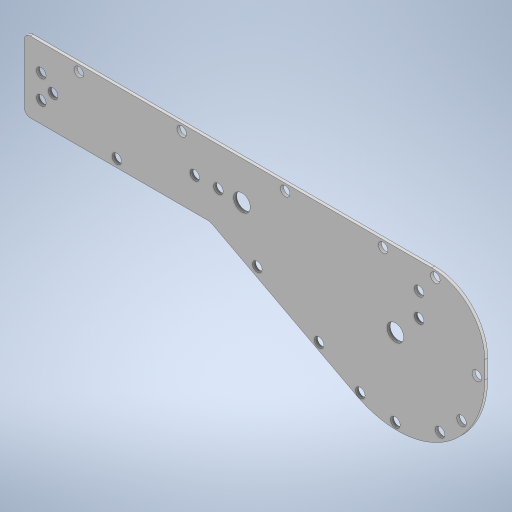
# Autodesk Inventor part: intake sled v5
Saved by Autodesk Inventor 2023.4 (Build 274418000, 418)
## iProperties
Created: 2023-12-16
Part Number: intake sled v5
Material: Generic
Document SubType Name: Modeling
Designer: Meer
Density: 1 g/cm^3
Appearance: Default
Author: Meer
Autodesk Inventor part; units mm, degrees
ref_plane "YZ Plane" through (0, 0, 0) normal (1, 0, 0) x (0, 1, 0)
ref_plane "XZ Plane" through (0, 0, 0) normal (0, 1, 0) x (-1, 0, 0)
ref_plane "XY Plane" through (0, 0, 0) normal (0, 0, 1) x (1, 0, 0)
sketch "Sketch1" plane through (0, 0, 0) normal (0, 0, 1) x (1, 0, 0)
  line L0 (0, 0) -> (247.65, 0)
  line L1 (247.65, 0) -> (247.65, 38.1)
  line L2 (247.65, 38.1) -> (0, 38.1)
  line L3 (0, 38.1) -> (0, 0)
  line L4 (286.1616, 0) -> (255.1962, 0)
  line L5 (255.1962, 0) -> (255.1962, 12.7)
  line L6 (255.1962, 12.7) -> (286.1616, 12.7)
  line L7 (286.1616, 12.7) -> (286.1616, 0)
  line L8 (247.65, 12.7) -> (200.66, 12.7)
  circle A0 centre (200.6294, 0) radius 47.0206
  line L9 (16.2468, 38.1) -> (16.2468, 12.7)
  line L10 (16.2468, 12.7) -> (155.3565, 12.7)
  line L11 (0, 12.7) -> (17.7951, 12.7)
  line L12 (179.5891, -42.0504) -> (75.8552, 12.7)
  point P0 (99.9175, 0)
  dimension "d0" = 247.65
  dimension "d1" = 38.1
  dimension "d2" = 12.7
  dimension "d3" = 30.9654
  dimension "d4" = 46.99
  dimension "d10" = 25.4
  constraints: 26 end point, 7 point on line, 5 perpendicular, 4 parallel, 3 point on circle, 2 horizontal, 1 centre point
  measures "d0" distance of L1.end L2.end
  measures "d1" distance of L0.end L1.end
  measures "d2" distance of L6.end L4.start
  measures "d3" distance of L5.end L6.end
  measures "d4" distance of L8.start L8.end
  measures "d10" distance of L9.start L9.end
extrude "Extrusion1" add sketch "Sketch1" along normal blind 1.5875 contours L3 L11 L10 L12 L0 | L12 L10 A0 L0 | L0 A0 L12 | L3 L2 L9 L11 | A0 L2 L0 | L0 A0 L12 | L10 L9 L2 A0 | A0 L8 L1 | L8 A0 L2 L1
fillet "Fillet1" radius 28.575 1 edges at (247.65, 38.1, 0.7937)
fillet "Fillet2" radius 3.175 1 edges at (0, 38.1, 0.7937)
fillet "Fillet4" radius 3.175 1 edges at (0, 0, 0.7937)
fillet "Fillet5" radius 5.08 1 edges at (99.9175, 0, 0.7937)
sketch "Sketch3" plane through (0, 0, 1.5875) normal (0, 0, 1) x (1, 0, 0)
  line L0 (9.1438, 0) -> (9.1438, 11.176)
  line L1 (9.1438, 11.176) -> (-0.0002, 11.176)
  circle A0 centre (9.1438, 11.176) radius 2.54
  line L2 (9.1438, 11.176) -> (9.1438, 23.876)
  circle A1 centre (9.1438, 23.876) radius 2.54
  line L3 (9.1438, 17.526) -> (15.4938, 17.526)
  circle A2 centre (15.4938, 17.526) radius 2.54
  line L4 (15.4938, 17.526) -> (91.6938, 17.526)
  circle A3 centre (91.6938, 17.526) radius 2.54
  line L5 (91.6938, 17.526) -> (104.3938, 17.526)
  circle A4 centre (104.3938, 17.526) radius 2.54
  line L6 (104.3938, 17.526) -> (117.0938, 17.526)
  circle A5 centre (117.0938, 17.526) radius 4.445
  line L7 (9.1438, 11.176) -> (212.3438, 11.176)
  line L8 (9.1438, 23.876) -> (212.3438, 23.876)
  circle A6 centre (212.3438, 23.876) radius 2.54
  circle A7 centre (212.3438, 11.176) radius 2.54
  circle A8 centre (125.3488, -8.3154) radius 2.54
  line L9 (125.3488, -8.3154) -> (158.5861, -26.9405)
  circle A9 centre (158.5861, -26.9405) radius 2.54
  line L10 (158.5861, -26.9405) -> (180.7442, -39.3573)
  circle A10 centre (180.7442, -39.3573) radius 2.54
  circle A11 centre (199.6056, -43.6188) radius 2.54
  circle A12 centre (223.6318, -36.189) radius 2.54
  circle A13 centre (235.2038, -25.0926) radius 2.54
  circle A14 centre (243.4585, 0) radius 2.54
  circle A15 centre (29.3464, 34.4582) radius 2.54
  circle A16 centre (84.6567, 34.4582) radius 2.54
  circle A17 centre (140.3584, 34.4582) radius 2.54
  circle A18 centre (192.9921, 34.4582) radius 2.54
  circle A19 centre (221.0918, 34.4582) radius 2.54
  circle A20 centre (49.7674, 4.225) radius 2.54
  arc A21 (101.0303, -0.5874) -> (98.6591, 0) centre (98.6591, -5.08) ccw projected
  line L11 (98.6591, 0) -> (199.6241, 0)
  line L12 (199.6241, 0) -> (199.6241, -1.778)
  circle A22 centre (199.6241, -1.778) radius 4.445
  point P0 (0, 0)
  point P1 (160.8019, -28.1822)
  point P2 (156.3703, -25.6989)
  point P3 (94.2338, 17.526)
  point P4 (89.1538, 17.526)
  point P5 (6.6038, 11.176)
  point P6 (9.1438, 8.636)
  point P7 (18.0338, 17.526)
  point P8 (12.9538, 17.526)
  point P9 (11.6838, 23.876)
  point P10 (9.1438, 21.336)
  dimension "d14" = 11.176
  dimension "d15" = 9.144
  dimension "d16" = 5.08
  dimension "d17" = 12.7
  dimension "d18" = 5.08
  dimension "d19" = 6.35
  dimension "d20" = 5.08
  dimension "d21" = 76.2
  dimension "d22" = 5.08
  dimension "d23" = 12.7
  dimension "d24" = 5.08
  dimension "d25" = 12.7
  dimension "d26" = 8.89
  dimension "d27" = 203.2
  dimension "d28" = 203.2
  dimension "d29" = 5.08
  dimension "d30" = 5.08
  dimension "d31" = 5.08
  dimension "d32" = 38.1
  dimension "d33" = 5.08
  dimension "d34" = 25.4
  dimension "d35" = 5.08
  dimension "d36" = 5.08
  dimension "d37" = 5.08
  dimension "d38" = 5.08
  dimension "d39" = 5.08
  dimension "d40" = 5.08
  dimension "d41" = 5.08
  dimension "d42" = 5.08
  dimension "d43" = 5.08
  dimension "d44" = 5.08
  dimension "d47" = 5.08
  dimension "d48" = 100.965
  dimension "d50" = 1.778
  dimension "d51" = 8.89
  constraints: 26 end point, 22 centre point, 12 coincident, 5 horizontal, 3 vertical, 2 point on line, 1 midpoint, 1 perpendicular
  measures "d14" distance of L0.start L0.end
  measures "d15" distance of L0.end L1.end
  measures "d16" diameter of A0
  measures "d17" distance of L2.start L2.end
  measures "d18" diameter of A1
  measures "d19" distance of L3.start L3.end
  measures "d20" diameter of A2
  measures "d21" distance of L4.start L4.end
  measures "d22" diameter of A3
  measures "d23" distance of L5.start L5.end
  measures "d24" diameter of A4
  measures "d25" distance of L6.start L6.end
  measures "d26" diameter of A5
  measures "d27" distance of L8.start L8.end
  measures "d28" distance of L2.start L7.end
  measures "d29" diameter of A6
  measures "d30" diameter of A7
  measures "d31" diameter of A8
  measures "d32" distance of L9.start L9.end
  measures "d33" diameter of A9
  measures "d34" distance of L10.start L10.end
  measures "d35" diameter of A10
  measures "d36" diameter of A11
  measures "d37" diameter of A12
  measures "d38" diameter of A13
  measures "d39" diameter of A14
  measures "d40" diameter of A15
  measures "d41" diameter of A16
  measures "d42" diameter of A17
  measures "d43" diameter of A18
  measures "d44" diameter of A19
  measures "d47" diameter of A20
  measures "d48" distance of L11.start L11.end
  measures "d50" distance of L12.start L12.end
  measures "d51" diameter of A22
extrude "Extrusion2" cut sketch "Sketch3" against normal blind 25.4
body "Solid1"
